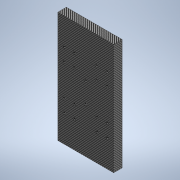
# Autodesk Inventor part: Placa6 Base3
Saved by Autodesk Inventor 2022 (Build 260153000, 153)
## iProperties
Created: 2021-11-08
Part Number: Placa6 Base3
Material: CFRP
Document SubType Name: Modeling
Designer: Samuel Gómez
Density: 1.43 g/cm^3
Appearance: Carbon Fiber
Author: Samuel Gómez
Autodesk Inventor part; units mm, degrees
ref_plane "YZ Plane" through (0, 0, 0) normal (1, 0, 0) x (0, 1, 0)
ref_plane "XZ Plane" through (0, 0, 0) normal (0, 1, 0) x (-1, 0, 0)
ref_plane "XY Plane" through (0, 0, 0) normal (0, 0, 1) x (1, 0, 0)
sketch "Boceto1" plane through (0, 0, 0) normal (0, 0, 1) x (1, 0, 0)
  line L0 (0, 0) -> (100, 0)
  line L1 (100, 0) -> (100, 200)
  line L2 (100, 200) -> (0, 200)
  line L3 (0, 200) -> (0, 0)
  dimension "d0" = 200
  dimension "d1" = 100
  constraints: 8 end point, 2 parallel, 1 horizontal, 1 perpendicular
  measures "d0" distance of L2.end L0.start
  measures "d1" distance of L0.start L0.end
extrude "Extrusión1" add sketch "Boceto1" along normal blind 15
sketch "Boceto2" plane through (0, 0, 15) normal (0, 0, 1) x (1, 0, 0)
  line L0 (100, 200) -> (0, 200) projected
  line L1 (50, 200) -> (50, 0) construction
  line L2 (0, 0) -> (100, 0) projected
  line L3 (50, 100) -> (0, 100) construction
  line L4 (50, 151.375) -> (30, 151.375) construction
  circle A0 centre (30, 151.375) radius 1.75
  line L5 (30, 151.375) -> (11.6, 151.375) construction
  circle A1 centre (11.6, 151.375) radius 1.75
  line L6 (30, 151.375) -> (30, 128.625) construction
  circle A2 centre (30, 128.625) radius 1.75
  line L7 (30, 128.625) -> (11.6, 128.625) construction
  line L8 (11.6, 128.625) -> (11.6, 151.375) construction
  circle A3 centre (11.6, 128.625) radius 1.75
  circle A4 centre (70, 151.375) radius 1.75
  circle A5 centre (88.4, 151.375) radius 1.75
  circle A6 centre (70, 128.625) radius 1.75
  circle A7 centre (88.4, 128.625) radius 1.75
  circle A8 centre (30, 48.625) radius 1.75
  circle A9 centre (11.6, 48.625) radius 1.75
  circle A10 centre (30, 71.375) radius 1.75
  circle A11 centre (11.6, 71.375) radius 1.75
  circle A12 centre (88.4, 48.625) radius 1.75
  circle A13 centre (70, 48.625) radius 1.75
  circle A14 centre (70, 71.375) radius 1.75
  circle A15 centre (88.4, 71.375) radius 1.75
  dimension "d5" = 51.375
  dimension "d6" = 20
  dimension "d7" = 3.5
  dimension "d8" = 18.4
  dimension "d9" = 3.5
  dimension "d10" = 3.5
  dimension "d11" = 22.75
  dimension "d12" = 3.5
  constraints: 16 centre point, 14 end point, 12 symmetric about line, 4 coincident, 4 horizontal, 3 midpoint, 1 perpendicular, 1 point on line, 1 vertical, 12 other
  measures "d5" distance between parallel lines of L3 L4
  measures "d6" distance of L4.start L4.end
  measures "d7" diameter of A0
  measures "d8" distance of L5.start L5.end
  measures "d9" diameter of A1
  measures "d10" diameter of A2
  measures "d11" distance of L5.start L6.end
  measures "d12" diameter of A3
extrude "Extrusión2" cut sketch "Boceto2" against normal up to surface (15 mm away)
sketch "Boceto3" plane through (0, 0, 15) normal (0, 0, 1) x (1, 0, 0)
  line L0 (0, 200) -> (0, 0) projected
  line L1 (0, 100) -> (100, 100) construction
  line L2 (100, 0) -> (100, 200) projected
  line L3 (100, 200) -> (0, 200) projected
  line L4 (50, 200) -> (50, 100) construction
  circle A0 centre (50, 118.25) radius 1.75
  circle A1 centre (50, 81.75) radius 1.75
  dimension "d15" = 3.5
  dimension "d16" = 18.25
  constraints: 4 end point, 4 midpoint, 2 centre point, 1 point on line, 1 symmetric about line, 1 other
  measures "d15" diameter of A0
  measures "d16" distance from line of L1 A0.centre
extrude "Extrusión3" cut sketch "Boceto3" against normal up to surface (15 mm away)
